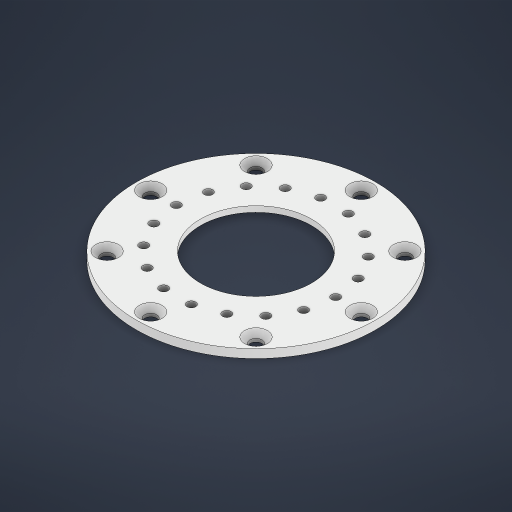
# Autodesk Inventor part: HousingLid
Saved by Autodesk Inventor 2024 (Build 280153000, 153)
## iProperties
Created: 2024-02-01
Part Number: HousingLid
Material: Generic
Document SubType Name: Modeling
Designer: avsar
Density: 1 g/cm^3
Appearance: Smooth - White
Author: avsar
Autodesk Inventor part; units mm, degrees
ref_plane "YZ Plane" through (0, 0, 0) normal (1, 0, 0) x (0, 1, 0)
ref_plane "XZ Plane" through (0, 0, 0) normal (0, 1, 0) x (-1, 0, 0)
ref_plane "XY Plane" through (0, 0, 0) normal (0, 0, 1) x (1, 0, 0)
sketch "Sketch1" plane through (0, 0, 0) normal (0, 1, 0) x (-1, 0, 0)
  circle A0 centre (0, 0) radius 42
  circle A1 centre (0, 0) radius 19.5
  circle A2 centre (0, -37) radius 2.1
  circle A3 centre (26.163, -26.163) radius 2.1
  circle A4 centre (37, 0) radius 2.1
  circle A5 centre (26.163, 26.163) radius 2.1
  circle A6 centre (0, 37) radius 2.1
  circle A7 centre (-26.163, 26.163) radius 2.1
  circle A8 centre (-37, 0) radius 2.1
  circle A9 centre (-26.163, -26.163) radius 2.1
  dimension "d0" = 84
  dimension "d1" = 39
  dimension "d2" = 4.2
  dimension "d3" = 37
  dimension "d6" = 360
  constraints: 10 centre point, 2 coincident, 1 vertical alignment, 17 other
  measures "d0" diameter of A0
  measures "d1" diameter of A1
  measures "d2" diameter of A2
  measures "d3" distance of A2.centre point (0, 0)
extrude "Extrusion1" add sketch "Sketch1" against normal blind 3
sketch "Sketch2" plane through (0, -3, 0) normal (0, -1, 0) x (1, 0, 0)
  circle A0 centre (0, 0) radius 24
  dimension "d10" = 48
  constraints: 1 centre point, 1 coincident
  measures "d10" diameter of A0
extrude "Extrusion2" cut sketch "Sketch2" against normal blind 1
hole "Hole1" at (37, 0, 0) at (26.163, 0, 26.163) at (0, 0, 37) at (-26.163, 0, 26.163) at (-37, 0, 0) at (-26.163, 0, -26.163) at (0, 0, -37) at (26.163, 0, -26.163) direction (0, -1, 0) diameter 4.2 end through all countersink diameter 8 countersink angle 90
sketch "Sketch3" plane through (0, 0, 0) normal (0, 1, 0) x (1, 0, 0)
  circle A0 centre (-4.8621, -27.5746) radius 1.5
  circle A1 centre (4.8621, -27.5746) radius 1.5
  circle A2 centre (14, -24.2487) radius 1.5
  circle A3 centre (21.4492, -17.9981) radius 1.5
  circle A4 centre (26.3114, -9.5766) radius 1.5
  circle A5 centre (28, 0) radius 1.5
  circle A6 centre (26.3114, 9.5766) radius 1.5
  circle A7 centre (21.4492, 17.9981) radius 1.5
  circle A8 centre (14, 24.2487) radius 1.5
  circle A9 centre (4.8621, 27.5746) radius 1.5
  circle A10 centre (-4.8621, 27.5746) radius 1.5
  circle A11 centre (-14, 24.2487) radius 1.5
  circle A12 centre (-21.4492, 17.9981) radius 1.5
  circle A13 centre (-26.3114, 9.5766) radius 1.5
  circle A14 centre (-28, 0) radius 1.5
  circle A15 centre (-26.3114, -9.5766) radius 1.5
  circle A16 centre (-21.4492, -17.9981) radius 1.5
  circle A17 centre (-14, -24.2487) radius 1.5
  line L0 (0, 0) -> (-4.8621, -27.5746) construction
  line L1 (0, 0) -> (0, -11.0753) construction
  dimension "d20" = 3
  dimension "d21" = 28
  dimension "d24" = 360
  dimension "d64" = 10
  constraints: 18 centre point, 4 end point, 1 coincident, 1 vertical, 37 other
  measures "d20" diameter of A0
  measures "d21" distance of L0.start A0.centre
  measures "d64" angle of L1 L0
extrude "Extrusion3" cut sketch "Sketch3" against normal through all
body "Solid1"
